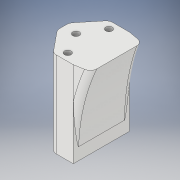
# Autodesk Inventor part: ArmBracket
Saved by Autodesk Inventor 2018 (Build 220112000, 112)
## iProperties
Created: 2019-01-19
Part Number: ArmBracket
Material: Generic
Document SubType Name: Modeling
Designer: anirudh
Density: 1 g/cm^3
Appearance: White
Author: anirudh
Autodesk Inventor part; units mm, degrees
ref_plane "YZ Plane" through (0, 0, 0) normal (1, 0, 0) x (0, 1, 0)
ref_plane "XZ Plane" through (0, 0, 0) normal (0, 1, 0) x (-1, 0, 0)
ref_plane "XY Plane" through (0, 0, 0) normal (0, 0, 1) x (1, 0, 0)
sketch "Sketch1" plane through (0, 0, 0) normal (0, 1, 0) x (-1, 0, 0)
  line L0 (0, 0) -> (10, 0)
  line L1 (10, -28) -> (0, -28)
  line L2 (0, -28) -> (0, 0)
  line L3 (19, -14) -> (19, -11)
  line L4 (19, -11) -> (19, -17)
  line L5 (10, 0) -> (19, -11)
  line L6 (19, -17) -> (10, -28)
  line L7 (0, 0) -> (6.5, 0)
  circle A0 centre (6.5, -3.75) radius 1.65
  circle A1 centre (6.5, -24.25) radius 1.65
  dimension "d3" = 3
  dimension "d5" = 6.5
  dimension "d10" = 3.3
  dimension "d11" = 3.3
  constraints: 16 end point, 2 centre point, 2 point on line, 1 horizontal, 1 parallel
  measures "d3" distance of L3.start L3.end
  measures "d5" distance of L0.start L7.end
  measures "d10" diameter of A0
  measures "d11" diameter of A1
extrude "Extrusion1" add sketch "Sketch1" along normal blind 42.672
sketch "Sketch2" plane through (0, 42.672, 0) normal (0, 1, 0) x (1, 0, 0)
  line L0 (-10, 0) -> (0, 0)
  circle A0 centre (-12.65, 14) radius 1.65
  point P0 (-19, 11)
  point P1 (0, 28)
  point P2 (-10, 28)
  point P3 (-19, 17)
  point P4 (-6.5, 24.25)
  dimension "d15" = 3.3
  constraints: 2 end point, 1 centre point, 1 horizontal
  measures "d15" diameter of A0
extrude "Extrusion2" cut sketch "Sketch2" against normal blind 12.7
sketch "Sketch3" plane through (0, 0, -28) normal (0, 0, -1) x (-1, 0, 0)
  line L0 (10, 42.672) -> (0, 42.672) projected
  line L1 (0, 42.672) -> (-7.62, 42.672)
  line L2 (0, 42.672) -> (0, 0)
  line L3 (0, 0) -> (0, 42.672) projected
  arc A0 (0, 6.0314) -> (-7.62, 42.672) centre (-106.4038, 3.0157) ccw
  constraints: 4 end point, 2 point on circle, 1 centre point, 1 horizontal, 1 point on line, 1 vertical
extrude "Extrusion3" add sketch "Sketch3" against normal blind 28
sketch "Sketch5" plane through (0, 0, -28) normal (0, 0, -1) x (-1, 0, 0)
  line L0 (19, 0) -> (10, 0) projected
  arc A0 (19, 42.672) -> (12.65, 7.0462) centre (135.5276, 3.5231) ccw
  line L1 (19, 0) -> (19, 42.672) projected
  line L2 (19, 42.672) -> (19, 0)
  line L3 (19, 0) -> (12.65, 0)
  line L4 (12.65, 7.0462) -> (12.65, 0)
  point P0 (0, 0)
  constraints: 6 end point, 2 point on circle, 2 vertical, 1 centre point, 1 point on line
extrude "Extrusion4" cut sketch "Sketch5" against normal blind 28
sketch "Sketch6" plane through (0, 42.672, 0) normal (0, 1, 0) x (1, 0, 0)
  line L0 (-10, 0) -> (7.62, 0) projected
  line L1 (0, 0) -> (7.62, 0)
  line L2 (-10, 28) -> (7.62, 28) projected
  line L3 (0, 28) -> (7.62, 28)
  line L4 (0, 0) -> (7.62, 0)
  arc A0 (7.62, 1.3039) -> (0, 0) centre (63.8048, -349.9581) ccw
  arc A1 (0, 28) -> (7.62, 26.6961) centre (63.8048, 377.9581) ccw
  line L5 (0, 0) -> (7.62, 0)
  line L6 (7.62, 28) -> (7.62, 0) projected
  line L7 (7.62, 0) -> (7.62, 1.3039)
  line L8 (7.62, 26.6961) -> (7.62, 28)
  line L9 (7.62, 28) -> (0, 28)
  constraints: 14 end point, 4 point on circle, 4 point on line, 3 collinear, 2 centre point, 2 horizontal, 1 perpendicular
extrude "Extrusion5" cut sketch "Sketch6" against normal blind 45.4625
fillet "Fillet3" radius 3.175 8 edges at (2.1549, 24.5337, -0.386) (2.1549, 24.5337, -27.614) (-10, 21.336, 0) (-14.5069, 25.094, -5.5084) (-12.65, 3.5231, -3.2389) (-14.5069, 25.094, -22.4916) (-12.65, 3.5231, -24.7611) (-10, 21.336, -28)
body "Solid1"
